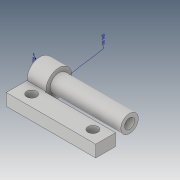
# Autodesk Inventor part: Cerniera 6
Saved by Autodesk Inventor 2019 (Build 230136000, 136)
## iProperties
Created: 2019-06-18
Part Number: Cerniera 6
Material: Generic
Document SubType Name: Modeling
Designer: giacomo
Density: 1 g/cm^3
Appearance: Default
Author: giacomo
Autodesk Inventor part; units mm, degrees
sketch "Sketch1" plane through (0, 0, 0) normal (0, 1, 0) x (-1, 0, 0)
  line L0 (16.1753, 16.3636) -> (-28.8247, 16.3636)
  line L1 (-28.8247, 16.3636) -> (-28.8247, 6.3636)
  line L2 (16.1753, 6.3636) -> (16.1753, 16.3636)
  line L3 (-17.8247, 6.3636) -> (-17.8247, 1.3636)
  line L4 (-17.8247, 1.3636) -> (5.1753, 1.3636)
  line L5 (5.1753, 1.3636) -> (5.1753, 6.3636)
  line L6 (-28.8247, 6.3636) -> (-17.8247, 6.3636)
  line L7 (5.1753, 6.3636) -> (16.1753, 6.3636)
  point P0 (0, 0)
  dimension "d4" = 45
  dimension "d5" = 5
  dimension "d6" = 5
  dimension "d7" = 11
  dimension "d8" = 11
  dimension "d9" = 23
  dimension "d10" = 10
  constraints: 16 end point, 4 parallel, 1 horizontal, 1 perpendicular
  measures "d4" distance of L0.start L0.end
  measures "d5" distance of L4.end L5.end
  measures "d6" distance of L3.start L3.end
  measures "d7" distance of L1.end L3.start
  measures "d8" distance of L5.end L2.start
  measures "d9" distance of L3.end L4.end
  measures "d10" distance of L2.start L0.start
extrude "Extrusion1" add sketch "Sketch1" along normal blind 6
sketch "Sketch4" plane through (17.8247, 0, 6.3636) normal (1, 0, 0) x (0, 0, -1)
  circle A0 centre (7, 6.5) radius 6.5
  line L0 (0, 6) -> (5, 6) projected
  line L1 (0, 0) -> (0, 6) projected
  line L2 (0, 0) -> (5, 0) projected
  point P0 (6.3636, 0)
  dimension "d20" = 13
  dimension "d36" = 7
  constraints: 1 centre point, 1 tangent
  measures "d20" diameter of A0
  measures "d36" distance from line of L1 A0.centre
extrude "Extrusion4" add sketch "Sketch4" against normal up to surface (23 mm away)
fillet "Fillet1" radius 12 2 edges at (6.3247, 0.3153, 1.3636) (6.3247, 0, 1.3636)
sketch "Sketch5" plane through (17.8247, 0, 6.3636) normal (1, 0, 0) x (0, 0, -1)
  circle A0 centre (7, 6.5) radius 6.5 projected
  circle A1 centre (7, 6.5) radius 2.5
  point P0 (6.3636, 0)
  point P1 (0.5193, 6)
  point P2 (6.2227, 0.0466)
  dimension "d27" = 5
  constraints: 1 centre point, 1 coincident
  measures "d27" diameter of A1
extrude "Extrusion5" cut sketch "Sketch5" against normal through all contours A1
ref_plane "Work Plane1" through (17.8247, 6.5, -7.1364) normal (0, 0, 1) x (1, 0, 0)
sketch "Sketch6" plane through (0, 6, 0) normal (0, 1, 0) x (1, 0, 0)
  circle A0 centre (-9.0753, -10.6636) radius 2.5
  circle A1 centre (21.7247, -10.6636) radius 2.5
  line L0 (37.8247, 7.1364) -> (-25.1753, 7.1364) projected
  line L1 (28.8247, -16.3636) -> (28.8247, -6.3636) projected
  line L2 (-16.1753, -6.3636) -> (-16.1753, -16.3636) projected
  point P0 (0, 0)
  dimension "d33" = 5
  dimension "d34" = 5
  dimension "d35" = 17.8
  dimension "d37" = 17.8
  dimension "d38" = 7.1
  dimension "d39" = 30.8
  dimension "d40" = 7.1
  constraints: 2 centre point
  measures "d33" diameter of A0
  measures "d34" diameter of A1
  measures "d35" distance from line of L0 A1.centre
  measures "d37" distance from line of L0 A0.centre
  measures "d38" distance from line of L1 A1.centre
  measures "d39" distance of A0.centre A1.centre
  measures "d40" distance from line of L2 A0.centre
extrude "Extrusion6" cut sketch "Sketch6" against normal through all
ref_plane "Work Plane8" through (-5.1753, 5.9967, 5.3636) normal (0, 0.0005541, -0.9999998) x (-1, 0, 0)
ref_plane "Work Plane10" through (28.8247, 0, 6.3636) normal (0, 0, -1) x (-1, 0, 0)
sketch "Sketch11" plane through (17.8247, 0, 6.3636) normal (1, 0, 0) x (0, 0, -1)
  circle A0 centre (7, 6.5) radius 2.5 projected
  arc A1 (6.2227, 0.0466) -> (0.5193, 6) centre (7, 6.5) ccw projected
  line L0 (0, 6) -> (0.5193, 6) projected
  line L1 (0, 0) -> (0, 6) projected
  line L2 (0, 0) -> (2.2671, 0) projected
  arc A2 (2.2671, 0) -> (3.5275, 0.0664) centre (2.2671, 12) ccw projected
  arc A3 (6.2227, 0.0466) -> (3.5275, 0.0664) centre (4.7878, -11.8673) ccw projected
  point P0 (6.3636, 0)
ref_plane "Work Plane11" through (17.8247, 0, 6.3636) normal (1, 0, 0) x (0, 0, -1)
ref_plane "Work Plane12" through (-5.1753, 0, 6.3636) normal (-1, 0, 0) x (0, 0, 1)
extrude "Extrusion10" add sketch "Sketch11" against normal up to surface (45 mm away) from surface at 11
extrude "Extrusion11" cut sketch "Sketch11" against normal up to surface (23 mm away) from surface at 0
move faces "Move1" translate (-1.5, 0, 0) faces at (-5.1753, 3.7794, 3.8394)
move faces "Move2" translate (17.25, 0, 0) faces at (17.8247, 3.7794, 3.8394)
sketch "Sketch13" plane through (-6.6753, 0, 6.3636) normal (1, 0, 0) x (0, 0, -1)
  circle A0 centre (7, 6.5) radius 2.5 projected
  circle A1 centre (7, 6.5) radius 4.4
  point P0 (6.3636, 0)
  dimension "d78" = 8.8
  constraints: 1 centre point
  measures "d78" diameter of A1
extrude "Extrusion13" add sketch "Sketch13" along normal up to surface (35.5 mm away)
body "Solid1"
